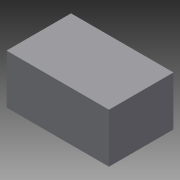
# Autodesk Inventor part: BIN
Saved by Autodesk Inventor 2015 (Build 190159000, 159)
## iProperties
Created: 2015-02-01
Part Number: BIN
Material: Generic
Document SubType Name: Modeling
Designer: chapale16
Density: 1 g/cm^3
Appearance: Default
Author: chapale16
Autodesk Inventor part; units mm, degrees
ref_plane "YZ Plane" through (0, 0, 0) normal (1, 0, 0) x (0, 1, 0)
ref_plane "XZ Plane" through (0, 0, 0) normal (0, 1, 0) x (-1, 0, 0)
ref_plane "XY Plane" through (0, 0, 0) normal (0, 0, 1) x (1, 0, 0)
sketch "Sketch1" plane through (0, 0, 0) normal (0, 1, 0) x (-1, 0, 0)
  line L0 (0, 0) -> (-685.8, 0)
  line L1 (-685.8, 0) -> (-685.8, -431.8)
  line L2 (-685.8, -431.8) -> (0, -431.8)
  line L3 (0, -431.8) -> (0, 0)
  dimension "d0" = 685.8
  dimension "d1" = 431.8
  constraints: 8 end point, 2 parallel, 1 horizontal, 1 perpendicular
  measures "d0" distance of L2.end L1.end
  measures "d1" distance of L1.end L0.end
extrude "Extrusion1" add sketch "Sketch1" along normal blind 330.2
body "Solid1"
